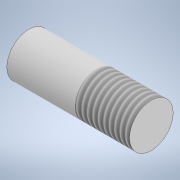
# Autodesk Inventor part: Шпилька
Saved by Autodesk Inventor 2021 (Build 250183000, 183)
## iProperties
Created: 2023-05-18
Part Number: Шпилька
Material: Типовые
Document SubType Name: Modeling
Designer: gdevc
Density: 1 g/cm^3
Appearance: По умолчанию
Author: gdevc
Autodesk Inventor part; units mm, degrees
ref_plane "YZ Plane" through (0, 0, 0) normal (1, 0, 0) x (0, 1, 0)
ref_plane "XZ Plane" through (0, 0, 0) normal (0, 1, 0) x (-1, 0, 0)
ref_plane "XY Plane" through (0, 0, 0) normal (0, 0, 1) x (1, 0, 0)
sketch "Эскиз1" plane through (0, 0, 0) normal (0, 0, 1) x (1, 0, 0)
  line L0 (0, 0) -> (0, 8)
  line L1 (0, 8) -> (45, 8)
  line L2 (45, 8) -> (45, 0)
  line L3 (0, 0) -> (45, 0)
  dimension "d0" = 45
  dimension "d1" = 16
  constraints: 8 end point, 2 vertical, 1 horizontal, 1 perpendicular
  measures "d0" distance of L0.end L1.end
  measures "d1" diameter of L1 L3
revolve "Вращение1" add sketch "Эскиз1" angle 360 about axis through (0, 0, 0) along (1, 0, 0)
thread "Резьба1" size "M16x2" class "6g" standard "ANSI Metric M Profile" length 20
